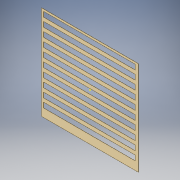
# Autodesk Inventor part: Front door
Saved by Autodesk Inventor 2018 (Build 220112000, 112)
## iProperties
Created: 2019-05-15
Part Number: Front door
Material: Generic
Document SubType Name: Modeling
Designer: 10043883
Density: 1 g/cm^3
Appearance: Wheat
Author: 10043883
Autodesk Inventor part; units mm, degrees
ref_plane "YZ Plane" through (0, 0, 0) normal (1, 0, 0) x (0, 1, 0)
ref_plane "XZ Plane" through (0, 0, 0) normal (0, 1, 0) x (-1, 0, 0)
ref_plane "XY Plane" through (0, 0, 0) normal (0, 0, 1) x (1, 0, 0)
sketch "Sketch1" plane through (0, 0, 0) normal (0, 0, 1) x (1, 0, 0)
  point P0 (0, 0)
sketch "Sketch2" plane through (0, 0, 0) normal (0, 0, 1) x (1, 0, 0)
  line L0 (-9271, -9017) -> (9271, -9017)
  line L1 (9271, -9017) -> (9271, 9017)
  line L2 (9271, 9017) -> (-9271, 9017)
  line L3 (-9271, 9017) -> (-9271, -9017)
  line L4 (-9271, -9017) -> (9271, 9017) construction
  line L5 (9271, -9017) -> (-9271, 9017) construction
  point P0 (0, 0)
  point P1 (-3003.2817, -9017)
  point P2 (-3003.2817, -2921)
  point P3 (3003.2817, -2921)
  point P4 (3003.2817, -9017)
  dimension "d0" = 18542
  dimension "d1" = 18034
  dimension "d2" = 6096
  constraints: 12 end point, 4 point on line, 2 midpoint, 2 parallel, 1 horizontal, 1 perpendicular
  measures "d0" distance of L2.end L1.end
  measures "d1" distance of L1.end L0.end
  measures "d2" distance of point (-3003.282, -9017) point (-3003.282, -2921)
extrude "Extrusion1" add sketch "Sketch2" along normal blind 25.4
sketch "Sketch3" plane through (0, 0, 25.4) normal (0, 0, 1) x (1, 0, 0)
  line L0 (-8892.2941, 8624.2343) -> (8699.9025, 8624.2343)
  line L1 (8699.9025, 8624.2343) -> (8699.9025, 7655.501)
  line L2 (8699.9025, 7655.501) -> (-8892.2941, 7655.501)
  line L3 (-8892.2941, 7655.501) -> (-8892.2941, 8624.2343)
  line L4 (8699.9025, 5979.101) -> (-8892.2941, 5979.101)
  line L5 (-8892.2941, 6947.8343) -> (8699.9025, 6947.8343)
  line L6 (-8892.2941, 5979.101) -> (-8892.2941, 6947.8343)
  line L7 (8699.9025, 6947.8343) -> (8699.9025, 5979.101)
  line L8 (8699.9025, 4302.701) -> (-8892.2941, 4302.701)
  line L9 (-8892.2941, 5271.4343) -> (8699.9025, 5271.4343)
  line L10 (-8892.2941, 4302.701) -> (-8892.2941, 5271.4343)
  line L11 (8699.9025, 5271.4343) -> (8699.9025, 4302.701)
  line L12 (8699.9025, 2626.301) -> (-8892.2941, 2626.301)
  line L13 (-8892.2941, 3595.0343) -> (8699.9025, 3595.0343)
  line L14 (-8892.2941, 2626.301) -> (-8892.2941, 3595.0343)
  line L15 (8699.9025, 3595.0343) -> (8699.9025, 2626.301)
  line L16 (8699.9025, 949.901) -> (-8892.2941, 949.901)
  line L17 (-8892.2941, 1918.6343) -> (8699.9025, 1918.6343)
  line L18 (-8892.2941, 949.901) -> (-8892.2941, 1918.6343)
  line L19 (8699.9025, 1918.6343) -> (8699.9025, 949.901)
  line L20 (8699.9025, -726.499) -> (-8892.2941, -726.499)
  line L21 (-8892.2941, 242.2343) -> (8699.9025, 242.2343)
  line L22 (-8892.2941, -726.499) -> (-8892.2941, 242.2343)
  line L23 (8699.9025, 242.2343) -> (8699.9025, -726.499)
  line L24 (8699.9025, -2402.899) -> (-8892.2941, -2402.899)
  line L25 (-8892.2941, -1434.1657) -> (8699.9025, -1434.1657)
  line L26 (-8892.2941, -2402.899) -> (-8892.2941, -1434.1657)
  line L27 (8699.9025, -1434.1657) -> (8699.9025, -2402.899)
  line L28 (8699.9025, -4079.299) -> (-8892.2941, -4079.299)
  line L29 (-8892.2941, -3110.5657) -> (8699.9025, -3110.5657)
  line L30 (-8892.2941, -4079.299) -> (-8892.2941, -3110.5657)
  line L31 (8699.9025, -3110.5657) -> (8699.9025, -4079.299)
  line L32 (8699.9025, -5755.699) -> (-8892.2941, -5755.699)
  line L33 (-8892.2941, -4786.9657) -> (8699.9025, -4786.9657)
  line L34 (-8892.2941, -5755.699) -> (-8892.2941, -4786.9657)
  line L35 (8699.9025, -4786.9657) -> (8699.9025, -5755.699)
  line L36 (8699.9025, -7432.099) -> (-8892.2941, -7432.099)
  line L37 (-8892.2941, -6463.3657) -> (8699.9025, -6463.3657)
  line L38 (-8892.2941, -7432.099) -> (-8892.2941, -6463.3657)
  line L39 (8699.9025, -6463.3657) -> (8699.9025, -7432.099)
  point P0 (0, 0)
  dimension "d7" = 1676.4
  constraints: 80 end point, 2 parallel, 1 collinear, 1 horizontal, 1 perpendicular, 1 vertical, 71 other
  measures "d7" distance of L1.end L4.start
extrude "Extrusion2" cut sketch "Sketch3" against normal through all
body "Solid1"
